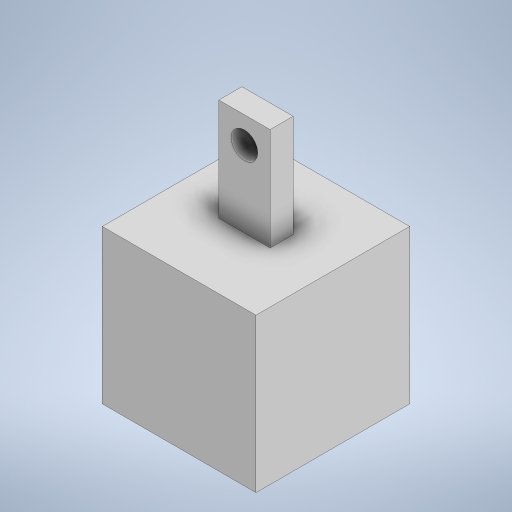
# Autodesk Inventor part: ObjectCube
Saved by Autodesk Inventor 2023 (Build 270158000, 158)
## iProperties
Created: 2023-10-26
Part Number: ObjectCube
Material: Generic
Document SubType Name: Modeling
Designer: Mustapha
Density: 1 g/cm^3
Appearance: Default
Author: Mustapha
Autodesk Inventor part; units mm, degrees
ref_plane "YZ Plane" through (0, 0, 0) normal (1, 0, 0) x (0, 1, 0)
ref_plane "XZ Plane" through (0, 0, 0) normal (0, 1, 0) x (-1, 0, 0)
ref_plane "XY Plane" through (0, 0, 0) normal (0, 0, 1) x (1, 0, 0)
sketch "Sketch1" plane through (0, 0, 0) normal (0, 1, 0) x (-1, 0, 0)
  line L0 (0, 0) -> (30, 0)
  line L1 (30, 0) -> (30, -30)
  line L2 (30, -30) -> (0, -30)
  line L3 (0, -30) -> (0, 0)
  dimension "d0" = 30
  dimension "d1" = 30
  constraints: 8 end point, 2 parallel, 1 horizontal, 1 perpendicular
  measures "d0" distance between parallel lines of L2 L0
  measures "d1" distance of L1.end L2.end
extrude "Extrusion1" add sketch "Sketch1" along normal blind 30
sketch "Sketch2" plane through (0, 30, 0) normal (0, 1, 0) x (1, 0, 0)
  line L0 (-20, 17.25) -> (-10, 17.25)
  line L1 (-10, 17.25) -> (-10, 12.75)
  line L2 (-10, 12.75) -> (-20, 12.75)
  line L3 (-20, 12.75) -> (-20, 17.25)
  line L4 (-20, 17.25) -> (-10, 12.75) construction
  line L5 (-10, 17.25) -> (-20, 12.75) construction
  line L6 (-30, 30) -> (-30, 0) projected
  line L7 (-30, 0) -> (0, 0) projected
  point P0 (-15, 15)
  point P1 (-30, 15)
  dimension "d4" = 15
  dimension "d5" = 15
  dimension "d6" = 10
  dimension "d7" = 4.5
  constraints: 12 end point, 3 midpoint, 2 parallel, 1 horizontal, 1 perpendicular
  measures "d4" distance of point (-30, 15) point (-15, 15)
  measures "d5" distance from line of L7 point (-15, 15)
  measures "d6" distance between parallel lines of L1 L3
  measures "d7" distance between parallel lines of L0 L2
extrude "Extrusion2" add sketch "Sketch2" along normal blind 20
sketch "Sketch3" plane through (-20, 30, -12.75) normal (0, 0, 1) x (1, 0, 0)
  circle A0 centre (5, 14.8617) radius 2.6
  point P0 (20, -30)
  dimension "d10" = 5.2
  constraints: 1 centre point
  measures "d10" diameter of A0
extrude "Extrusion3" cut sketch "Sketch3" against normal blind 20
body "Solid1"
